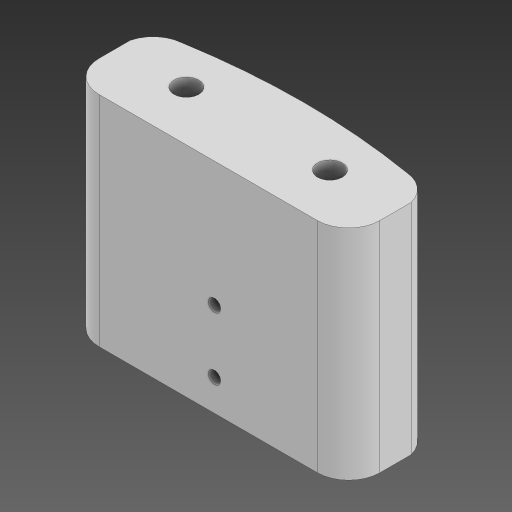
# Autodesk Inventor part: handle mount
Saved by Autodesk Inventor 2023 (Build 270158000, 158)
## iProperties
Created: 2025-06-22
Part Number: handle mount
Material: Типовые
Document SubType Name: Modeling
Designer: daa
Density: 1 g/cm^3
Appearance: По умолчанию
Author: daa
Autodesk Inventor part; units mm, degrees
ref_plane "YZ Plane" through (0, 0, 0) normal (1, 0, 0) x (0, 1, 0)
ref_plane "XZ Plane" through (0, 0, 0) normal (0, 1, 0) x (-1, 0, 0)
ref_plane "XY Plane" through (0, 0, 0) normal (0, 0, 1) x (1, 0, 0)
sketch "Эскиз1" plane through (0, 0, 0) normal (0, 1, 0) x (-1, 0, 0)
  line L0 (-3.5, 12) -> (-38.5, 12)
  arc A0 (1.5, 7) -> (-3.5, 12) centre (-3.5, 7) ccw
  arc A1 (-38.5, 12) -> (-43.5, 7) centre (-38.5, 7) ccw
  line L1 (-3, -1.8) -> (-39, -1.8)
  line L2 (-43.5, 7) -> (-43.5, 2)
  line L3 (2, -3.3) -> (-49, -3.3)
  arc A2 (-39, -1.8) -> (-3, -1.8) centre (-21, 105.3667) ccw
  line L4 (1.5, 7) -> (1.5, 2)
  arc A3 (-3, -1.8) -> (1.5, 2) centre (-3.357, 3.1872) ccw
  arc A4 (-43.5, 2) -> (-39, -1.8) centre (-38.643, 3.1872) ccw
  point P0 (-43, 12)
  point P1 (-21.5, -3.3)
  point P2 (1.5, 4.5)
  point P3 (-39, -1.8)
  point P4 (-39, -1.8)
  point P5 (-21.5, -3.3)
  point P6 (-20.5, -3.3)
  dimension "d5" = 5
  dimension "d13" = 5
  dimension "d17" = 13.8
  dimension "d20" = 15.3
  dimension "d55" = 108.6678
  dimension "d56" = 36
  dimension "d57" = 5
  dimension "d58" = 4.5
  dimension "d59" = 45
  dimension "d60" = 5
  dimension "d61" = 5
  constraints: 11 point on circle, 10 end point, 5 centre point, 3 horizontal, 2 tangent, 2 vertical, 1 equal radius, 1 midpoint, 1 point on line
  measures "d5" radius of A0
  measures "d13" distance of L2.start L2.end
  measures "d17" distance between parallel lines of L1 L0
  measures "d20" distance from line of point (-21.5, -3.3) L0
  measures "d55" radius of A2
  measures "d56" distance of L1.start L1.end
  measures "d57" distance of L4.start L4.end
  measures "d58" distance from line of L1.start L4
  measures "d59" distance from line of L2 point (1.5, 4.5)
  measures "d60" radius of A3
  measures "d61" radius of A4
extrude "Выдавливание1" add sketch "Эскиз1" along normal blind 35
sketch "Эскиз2" plane through (0, 0, 0) normal (0, -1, 0) x (1, 0, 0)
  circle A0 centre (32.5, 4.35) radius 2
  circle A1 centre (9.5, 4.35) radius 2
  line L0 (3.5, 12) -> (38.5, 12) projected
  line L1 (-1.5, 2) -> (-1.5, 7) projected
  point P0 (0, 0)
  dimension "d21" = 4
  dimension "d22" = 4
  dimension "d24" = 7.65
  dimension "d25" = 7.65
  dimension "d26" = 23
  dimension "d62" = 11
  constraints: 2 centre point
  measures "d21" diameter of A0
  measures "d22" diameter of A1
  measures "d24" distance from line of A1.centre L0
  measures "d25" distance from line of A0.centre L0
  measures "d26" distance of A1.centre A0.centre
  measures "d62" distance from line of L1 A1.centre
extrude "Выдавливание2" cut sketch "Эскиз2" against normal blind 5.5
sketch "Эскиз3" plane through (0, 35, 0) normal (0, 1, 0) x (1, 0, 0)
  circle A0 centre (9.5, -4) radius 2
  line L0 (3.5, -12) -> (38.5, -12) projected
  circle A1 centre (32.5, -4) radius 2
  line L1 (43.5, -7) -> (43.5, -2) projected
  line L2 (-1.5, -2) -> (-1.5, -7) projected
  point P0 (0, 0)
  point P1 (31.5, -4)
  point P2 (43.5, -4.5)
  dimension "d29" = 4
  dimension "d32" = 8
  dimension "d33" = 4
  dimension "d34" = 8
  dimension "d36" = 23
  dimension "d64" = 11
  constraints: 2 centre point, 1 midpoint
  measures "d29" diameter of A0
  measures "d32" distance from line of L0 A0.centre
  measures "d33" diameter of A1
  measures "d34" distance from line of L0 A1.centre
  measures "d36" distance of A0.centre A1.centre
  measures "d64" distance from line of A0.centre L2
extrude "Выдавливание3" cut sketch "Эскиз3" against normal blind 5.5
sketch "Эскиз4" plane through (0, 0, 0) normal (0, -1, 0) x (1, 0, 0)
  circle A0 centre (21, 4.35) radius 1.75
  line L0 (43.5, 7) -> (43.5, 2) projected
  line L1 (3.5, 12) -> (38.5, 12) projected
  point P0 (0, 0)
  dimension "d39" = 3.5
  dimension "d40" = 22.5
  dimension "d41" = 7.65
  constraints: 1 centre point
  measures "d39" diameter of A0
  measures "d40" distance from line of L0 A0.centre
  measures "d41" distance from line of A0.centre L1
extrude "Выдавливание4" cut sketch "Эскиз4" against normal blind 20
sketch "Эскиз5" plane through (3.5, 0, 12) normal (0, 0, 1) x (1, 0, 0)
  circle A0 centre (18.5, 5) radius 1
  circle A1 centre (18.5, 15) radius 1
  line L0 (35, 0) -> (35, 35) projected
  line L1 (0, 0) -> (35, 0) projected
  point P0 (-3.5, 0)
  dimension "d44" = 2
  dimension "d45" = 2
  dimension "d46" = 16.5
  dimension "d47" = 16.5
  dimension "d48" = 10
  dimension "d49" = 5
  constraints: 2 centre point
  measures "d44" diameter of A0
  measures "d45" diameter of A1
  measures "d46" distance from line of A0.centre L0
  measures "d47" distance from line of A1.centre L0
  measures "d48" distance of A1.centre A0.centre
  measures "d49" distance from line of L1 A0.centre
extrude "Выдавливание5" cut sketch "Эскиз5" against normal through all
fillet "Сопряжение3" radius 0.5 4 edges at (22.5628, 14.1734, -3.2899) (22.5618, 15.8272, -3.2899) (22.5628, 4.1734, -3.2899) (22.5618, 5.8272, -3.2899)
